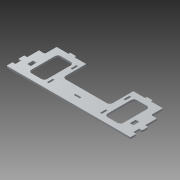
# Autodesk Inventor part: Bulkhead 25083113
Saved by Autodesk Inventor 2015 (Build 190159000, 159)
## iProperties
Created: 2011-09-23
Part Number: Bulkhead 25083113
Document SubType Name: Modeling
Designer: user
Density: 1 g/cm^3
Material: Generic
Appearance: Steel Blue
Author: user
Autodesk Inventor part; units mm, degrees
ref_plane "YZ Plane" through (0, 0, 0) normal (1, 0, 0) x (0, 1, 0)
ref_plane "XZ Plane" through (0, 0, 0) normal (0, 1, 0) x (-1, 0, 0)
ref_plane "XY Plane" through (0, 0, 0) normal (0, 0, 1) x (1, 0, 0)
sketch "Sketch1" plane through (0, 0, 0) normal (0, 0, 1) x (1, 0, 0)
  line L0 (-40, 0) -> (-40, -35)
  line L1 (-35, -40) -> (35, -40)
  line L2 (40, -35) -> (40, 0)
  line L3 (104, -70) -> (-104, -70)
  line L4 (-60, 0) -> (-60, 3)
  line L5 (-60, 3) -> (-70, 3)
  line L6 (-70, 3) -> (-70, 0)
  line L7 (-90, 0) -> (-70, 0)
  line L8 (-60, 0) -> (-40, 0)
  line L9 (70, 0) -> (70, 3)
  line L10 (70, 3) -> (60, 3)
  line L11 (60, 3) -> (60, 0)
  line L12 (40, 0) -> (60, 0)
  line L13 (70, 0) -> (90, 0)
  arc A0 (-105, -69) -> (-104, -70) centre (-104, -69) ccw
  arc A1 (104, -70) -> (105, -69) centre (104, -69) ccw
  line L14 (-90, -40) -> (-84, -40)
  line L15 (-84, -40) -> (-84, -50)
  line L16 (90, -40) -> (84, -40)
  line L17 (84, -40) -> (84, -50)
  line L18 (-43.5, -10) -> (-46.5, -10)
  line L19 (-46.5, -10) -> (-46.5, -20)
  line L20 (-46.5, -20) -> (-43.5, -20)
  line L21 (-43.5, -20) -> (-43.5, -10)
  line L22 (43.5, -10) -> (46.5, -10)
  line L23 (46.5, -10) -> (46.5, -20)
  line L24 (46.5, -20) -> (43.5, -20)
  line L25 (43.5, -20) -> (43.5, -10)
  line L26 (-46.5, -50) -> (-43.5, -50)
  line L27 (-43.5, -50) -> (-43.5, -60)
  line L28 (-43.5, -60) -> (-46.5, -60)
  line L29 (-46.5, -60) -> (-46.5, -50)
  line L30 (43.5, -50) -> (46.5, -50)
  line L31 (46.5, -50) -> (46.5, -60)
  line L32 (46.5, -60) -> (43.5, -60)
  line L33 (43.5, -60) -> (43.5, -50)
  line L34 (-5, -53) -> (5, -53)
  line L35 (5, -53) -> (5, -56)
  line L36 (5, -56) -> (-5, -56)
  line L37 (-5, -56) -> (-5, -53)
  line L38 (-100, -40) -> (-100, -20)
  line L39 (-100, -20) -> (-92, -20)
  line L40 (-90, -40) -> (-90, -50)
  line L41 (90, -40) -> (90, -50)
  line L42 (90, -50) -> (84, -50)
  line L43 (100, -40) -> (100, -20)
  line L44 (100, -20) -> (92, -20)
  line L45 (90, -18) -> (90, 0)
  line L46 (-90, 0) -> (-90, -18)
  arc A2 (-92, -20) -> (-90, -18) centre (-92, -18) ccw
  arc A3 (90, -18) -> (92, -20) centre (92, -18) ccw
  line L47 (-90, -50) -> (-84, -50)
  line L48 (-100, -40) -> (-104, -40)
  line L49 (100, -40) -> (104, -40)
  arc A4 (-104, -40) -> (-105, -41) centre (-104, -41) ccw
  arc A5 (105, -41) -> (104, -40) centre (104, -41) ccw
  line L50 (-104, -50) -> (-100, -50)
  line L51 (-100, -50) -> (-100, -60)
  line L52 (-100, -60) -> (-104, -60)
  line L53 (-105, -69) -> (-105, -61)
  line L54 (-105, -49) -> (-105, -41)
  arc A6 (-104, -60) -> (-105, -61) centre (-104, -61) ccw
  arc A7 (-105, -49) -> (-104, -50) centre (-104, -49) ccw
  line L55 (104, -50) -> (100, -50)
  line L56 (100, -50) -> (100, -60)
  line L57 (100, -60) -> (104, -60)
  line L58 (105, -41) -> (105, -49)
  line L59 (105, -61) -> (105, -69)
  arc A8 (105, -61) -> (104, -60) centre (104, -61) ccw
  arc A9 (104, -50) -> (105, -49) centre (104, -49) ccw
  arc A10 (-40, -35) -> (-35, -40) centre (-35, -35) ccw
  arc A11 (35, -40) -> (40, -35) centre (35, -35) ccw
  line L60 (-73, -10) -> (-56, -10)
  line L61 (-51, -15) -> (-51, -55)
  line L62 (-56, -60) -> (-73, -60)
  line L63 (-78, -55) -> (-78, -15)
  line L64 (56, -10) -> (73, -10)
  line L65 (78, -15) -> (78, -55)
  line L66 (73, -60) -> (56, -60)
  line L67 (51, -55) -> (51, -15)
  arc A12 (-73, -10) -> (-78, -15) centre (-73, -15) ccw
  arc A13 (-51, -15) -> (-56, -10) centre (-56, -15) ccw
  arc A14 (-56, -60) -> (-51, -55) centre (-56, -55) ccw
  arc A15 (-78, -55) -> (-73, -60) centre (-73, -55) ccw
  arc A16 (56, -10) -> (51, -15) centre (56, -15) ccw
  arc A17 (78, -15) -> (73, -10) centre (73, -15) ccw
  arc A18 (73, -60) -> (78, -55) centre (73, -55) ccw
  arc A19 (51, -55) -> (56, -60) centre (56, -55) ccw
  point P0 (0, 0)
  point P1 (105, -70)
  point P2 (-105, -70)
  point P3 (-90, -20)
  point P4 (90, -20)
  point P5 (-105, -40)
  point P6 (105, -50)
  point P7 (-40, -40)
  point P8 (40, -40)
  dimension "d0" = 80
  dimension "d1" = 40
  dimension "d2" = 50
  dimension "d10" = 50
  dimension "d15" = 3
  dimension "d16" = 10
  dimension "d18" = 10
  dimension "d20" = 3
  dimension "d23" = 40
  dimension "d24" = 40
  dimension "d27" = 1
  dimension "d28" = 10
  dimension "d29" = 6
  dimension "d31" = 40
  dimension "d32" = 10
  dimension "d33" = 6
  dimension "d35" = 40
  dimension "d39" = 10
  dimension "d40" = 3
  dimension "d41" = 10
  dimension "d42" = 3
  dimension "d44" = 10
  dimension "d45" = 10
  dimension "d50" = 3
  dimension "d51" = 10
  dimension "d52" = 10
  dimension "d54" = 3
  dimension "d55" = 10
  dimension "d56" = 10
  dimension "d60" = 10
  dimension "d61" = 3
  dimension "d62" = 17
  dimension "d66" = 40
  dimension "d67" = 40
  dimension "d71" = 3.5
  dimension "d72" = 3.5
  dimension "d73" = 3.5
  dimension "d74" = 3.5
  dimension "d77" = 20
  dimension "d78" = 20
  dimension "d79" = 10
  dimension "d80" = 10
  dimension "d81" = 2
  dimension "d82" = 10
  dimension "d84" = 50
  dimension "d85" = 20
  dimension "d86" = 20
  dimension "d87" = 60
  dimension "d88" = 5
  dimension "d92" = 30
  dimension "d93" = 5
  dimension "d94" = 30
  dimension "d95" = 1
  dimension "d97" = 10
  dimension "d98" = 10
  dimension "d99" = 1
  dimension "d100" = 10
  dimension "d101" = 10
  dimension "d102" = 5
  dimension "d103" = 5
  dimension "d104" = 210
  dimension "d105" = 1
  dimension "d106" = 5
  dimension "d107" = 70
  constraints: 136 end point, 44 tangent, 40 point on circle, 31 parallel, 23 perpendicular, 20 centre point, 13 equal radius, 13 point on line, 11 horizontal, 5 collinear
  measures "d0" distance of point (-40, -40) point (40, -40)
  measures "d1" distance of point (40, -40) L2.end
  measures "d2" distance of L2.end L13.end
  measures "d10" distance of L7.start L0.start
  measures "d15" distance between parallel lines of L5 L7
  measures "d16" distance of L4.end L5.end
  measures "d18" distance of L9.end L10.end
  measures "d20" distance between parallel lines of L13 L10
  measures "d23" distance from line of point (0, 0) L1
  measures "d24" distance from line of point (0, 0) L2
  measures "d27" radius of A0
  measures "d28" distance of L14.end L15.end
  measures "d29" distance of L14.start L14.end
  measures "d31" distance between parallel lines of L8 L14
  measures "d32" distance of L16.end L17.end
  measures "d33" distance of L16.start L16.end
  measures "d35" distance between parallel lines of L12 L16
  measures "d39" distance of L20.end L18.start
  measures "d40" distance of L19.end L20.end
  measures "d41" distance between parallel lines of L8 L18
  measures "d42" distance of L22.start L22.end
  measures "d44" distance of L22.end L23.end
  measures "d45" distance between parallel lines of L12 L22
  measures "d50" distance of L27.end L28.end
  measures "d51" distance of L28.end L26.start
  measures "d52" distance between parallel lines of L3 L28
  measures "d54" distance of L31.end L32.end
  measures "d55" distance of L30.end L31.end
  measures "d56" distance between parallel lines of L3 L32
  measures "d60" distance of L35.end L36.end
  measures "d61" distance of L34.end L35.end
  measures "d62" distance between parallel lines of L3 L34
  measures "d66" distance of L7.start L14.start
  measures "d67" distance of L16.start L13.end
  measures "d71" distance between parallel lines of L2 L25
  measures "d72" distance between parallel lines of L0 L21
  measures "d73" distance between parallel lines of L0 L27
  measures "d74" distance between parallel lines of L33 L2
  measures "d77" distance between parallel lines of L7 L39
  measures "d78" distance of point (90, -20) L13.end
  measures "d79" distance of L43.end point (90, -20)
  measures "d80" distance of L38.end point (-90, -20)
  measures "d81" radius of A2
  measures "d82" distance between parallel lines of L38 L40
  measures "d84" distance between parallel lines of L3 L39
  measures "d85" distance between parallel lines of L46 L6
  measures "d86" distance between parallel lines of L45 L9
  measures "d87" distance from line of L11 point (0, 0)
  measures "d88" distance from line of point (0, 0) L37
  measures "d92" distance between parallel lines of L3 L48
  measures "d93" distance of L38.start point (-105, -40)
  measures "d94" distance between parallel lines of L3 L49
  measures "d95" radius of A4
  measures "d97" distance between parallel lines of L48 L50
  measures "d98" distance between parallel lines of L3 L52
  measures "d99" radius of A6
  measures "d100" distance between parallel lines of L49 L55
  measures "d101" distance between parallel lines of L57 L3
  measures "d102" distance between parallel lines of L51 L54
  measures "d103" distance of point (105, -50) L55.end
  measures "d104" distance between parallel lines of L53 L59
  measures "d105" radius of A8
  measures "d106" distance between parallel lines of L43 L58
  measures "d107" distance between parallel lines of L3 L13
extrude "Extrusion8" add sketch "Sketch1" along normal blind 3
body "Solid8"
